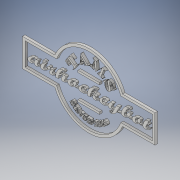
# Autodesk Inventor part: Emblem_script
Saved by Autodesk Inventor 2019.3 (Build 233278000, 278)
## iProperties
Created: 2020-09-20
Part Number: Emblem_script
Material: Generisch
Document SubType Name: Modeling
Designer: Nicolas Frick
Density: 1 g/cm^3
Appearance: Vorgabe
Author: Nicolas Frick
Autodesk Inventor part; units mm, degrees
(part 1 of 2)
ref_plane "YZ Plane" through (0, 0, 0) normal (1, 0, 0) x (0, 1, 0)
ref_plane "XZ Plane" through (0, 0, 0) normal (0, 1, 0) x (-1, 0, 0)
sketch "Skizze1" plane through (0, 0, 0) normal (0, 0, 1) x (1, 0, 0)
  line L0 (-50, 9) -> (-50, -9) construction
  line L1 (50, 9) -> (50, -9) construction
  line L2 (-50, -9) -> (-50, 9)
  line L3 (-50, 9) -> (-25.1982, 9)
  line L4 (25.1982, 9) -> (50, 9)
  line L5 (50, -9) -> (25.1982, -9)
  line L6 (-25.1982, -9) -> (-50, -9)
  line L7 (50, 9) -> (29.5255, 5.3146) construction
  arc A0 (25.1982, 9) -> (-25.1982, 9) centre (0, 0) ccw
  arc A1 (-25.1982, -9) -> (25.1982, -9) centre (0, 0) ccw
  line L8 (50, -12.5) -> (50, -9) construction
  line L9 (50, 9) -> (50, 12.5) construction
  line L10 (50, 9) -> (50, -9)
  point P0 (0, 0)
  dimension "d13" = 100
  dimension "d14" = 18
  constraints: 22 end point, 7 parallel, 4 point on circle, 2 centre point, 2 horizontal, 2 perpendicular, 1 coincident, 1 collinear
  measures "d13" distance of L0.end L1.end
  measures "d14" distance of L1.start L1.end
ref_plane "Arbeitsebene3" through (0, 0, 0) normal (0, 0, -1) x (-1, 0, 0)
sketch "Skizze3" plane through (0, 0, 0) normal (0, 0, -1) x (-1, 0, 0)
  line L0 (50, -12.5) -> (50, 12.5) construction
  line L1 (50, 12.5) -> (27.2718, 12.5) construction
  arc A0 (27.2718, 12.5) -> (-27.2718, 12.5) centre (0, 0) ccw construction
  line L2 (-27.2718, 12.5) -> (-50, 12.5) construction
  line L3 (-50, 12.5) -> (-50, -12.5) construction
  line L4 (-50, -12.5) -> (-27.2718, -12.5) construction
  arc A1 (-27.2718, -12.5) -> (27.2718, -12.5) centre (0, 0) ccw construction
  line L5 (27.2718, -12.5) -> (50, -12.5) construction
  line L6 (50, 9) -> (50, -9) projected
  line L7 (50, -9) -> (25.1982, -9) projected
  arc A2 (-25.1982, -9) -> (25.1982, -9) centre (0, 0) ccw projected
  line L8 (-25.1982, -9) -> (-50, -9) projected
  line L9 (-50, -9) -> (-50, 9) projected
  line L10 (-50, 9) -> (-25.1982, 9) projected
  arc A3 (25.1982, 9) -> (-25.1982, 9) centre (0, 0) ccw projected
  line L11 (25.1982, 9) -> (50, 9) projected
  line L12 (-26.5702, 11) -> (-52, 11)
  line L13 (-52, 11) -> (-52, -11)
  line L14 (-52, -11) -> (-26.5702, -11)
  arc A4 (-26.5702, -11) -> (26.5702, -11) centre (0, 0) ccw
  line L15 (26.5702, -11) -> (52, -11)
  line L16 (52, -11) -> (52, 11)
  line L17 (52, 11) -> (26.5702, 11)
  arc A5 (26.5702, 11) -> (-26.5702, 11) centre (0, 0) ccw
  dimension "d15" = 2
  constraints: 12 end point, 4 point on circle, 2 centre point, 7 other
  measures "d15" radial gap between concentric circles of A3 A5
ref_plane "Arbeitsebene2" through (0, 0, 3) normal (0, 0, 1) x (1, 0, 0)
sketch "Skizze4" plane through (0, 0, 3) normal (0, 0, 1) x (1, 0, 0)
  arc A0 (27.2718, 12.5) -> (-27.2718, 12.5) centre (0, 0) ccw construction
  arc A1 (14.0689, 14.5714) -> (-13.3793, 13.406) centre (0.8375, 2.3845) ccw construction
  line L0 (-50, 9) -> (-50, -9) projected
  line L1 (-48.0831, -3.7083) -> (51.9405, -3.7083) construction
  line L2 (-0.0067, -3.7083) -> (-47.5067, -3.7083) construction
  line L3 (-47.5067, -3.7083) -> (47.4933, -3.7083) construction
  arc A2 (-13.3793, -16.6178) -> (14.0689, -16.6178) centre (0.3448, -2.5459) ccw construction
  spline S0 degree 2 poles (-37.8675, -2.4944) (-39.3666, -3.3302) (-40.6602, -3.8343) (-41.2506, -3.8343) knots 0 0 0 1 2 2 2
  spline S1 degree 2 poles (-41.2506, -3.8343) (-42.7365, -3.8343) (-42.6502, -2.2953) knots 0 0 0 1 1 1
  spline S2 degree 2 poles (-42.6502, -2.2953) (-43.5855, -3.0847) (-45.171, -3.8343) (-46.0134, -3.8343) knots 0 0 0 1 2 2 2
  spline S3 degree 2 poles (-46.0134, -3.8343) (-46.836, -3.8343) (-47.9902, -2.9255) (-47.9902, -2.2622) knots 0 0 0 1 2 2 2
  spline S4 degree 2 poles (-47.9902, -2.2622) (-47.9902, -1.4396) (-46.4446, 0.0595) (-44.03, 0.9882) (-43.1013, 0.9882) knots 0 0 0 1 2 3 3 3
  spline S5 degree 2 poles (-43.1013, 0.9882) (-41.9272, 0.9882) (-41.4628, 0.3514) knots 0 0 0 1 1 1
  line L4 (-41.4628, 0.3514) -> (-39.5457, 0.975)
  line L5 (-39.5457, 0.975) -> (-39.0217, 0.975)
  line L6 (-39.0217, 0.975) -> (-39.8443, -0.637)
  spline S6 degree 2 poles (-39.8443, -0.637) (-40.4877, -1.8575) (-40.4877, -2.3086) knots 0 0 0 1 1 1
  spline S7 degree 2 poles (-40.4877, -2.3086) (-40.4877, -2.7796) (-39.9106, -2.7796) knots 0 0 0 1 1 1
  spline S8 degree 2 poles (-39.9106, -2.7796) (-39.5457, -2.7796) (-38.6635, -2.3219) (-37.8675, -1.8575) knots 0 0 0 1 2 2 2
  line L7 (-37.8675, -1.8575) -> (-37.8675, -2.4944)
  spline S9 degree 2 poles (-44.7265, -2.7929) (-43.7912, -2.7929) (-42.1328, -0.9156) (-42.1328, -0.1196) knots 0 0 0 1 2 2 2
  spline S10 degree 2 poles (-42.1328, -0.1196) (-42.1328, 0.1922) (-42.6038, 0.5372) (-42.9952, 0.5372) knots 0 0 0 1 2 2 2
  spline S11 degree 2 poles (-42.9952, 0.5372) (-43.9305, 0.5372) (-45.6088, -1.3401) (-45.6088, -2.1229) knots 0 0 0 1 2 2 2
  spline S12 degree 2 poles (-45.6088, -2.1229) (-45.6088, -2.4214) (-45.1112, -2.7929) (-44.7265, -2.7929) knots 0 0 0 1 2 2 2
  spline S13 degree 2 poles (-33.1444, -2.4944) (-35.3335, -3.8476) (-36.4214, -3.8476) knots 0 0 0 1 1 1
  spline S14 degree 2 poles (-36.4214, -3.8476) (-37.025, -3.8476) (-37.8476, -3.1245) (-37.8476, -2.5806) knots 0 0 0 1 2 2 2
  spline S15 degree 2 poles (-37.8476, -2.5806) (-37.8476, -1.4065) (-36.501, 0.6698) knots 0 0 0 1 1 1
  line L8 (-36.501, 0.6698) -> (-34.1195, 0.9617)
  line L9 (-34.1195, 0.9617) -> (-34.0068, 0.9617)
  line L10 (-34.0068, 0.9617) -> (-34.9421, -0.763)
  spline S16 degree 2 poles (-34.9421, -0.763) (-35.5258, -1.831) (-35.5258, -2.2887) knots 0 0 0 1 1 1
  spline S17 degree 2 poles (-35.5258, -2.2887) (-35.5258, -2.4678) (-35.2539, -2.6934) (-35.0482, -2.6934) knots 0 0 0 1 2 2 2
  spline S18 degree 2 poles (-35.0482, -2.6934) (-34.6834, -2.6934) (-33.9404, -2.3816) (-33.1444, -1.8575) knots 0 0 0 1 2 2 2
  line L11 (-33.1444, -1.8575) -> (-33.1444, -2.4944)
  spline S19 degree 2 poles (-33.3302, 3.111) (-33.3302, 1.7909) (-34.9885, 1.7909) knots 0 0 0 1 1 1
  spline S20 degree 2 poles (-34.9885, 1.7909) (-35.7978, 1.7909) (-36.3683, 2.0761) knots 0 0 0 1 1 1
  spline S21 degree 2 poles (-36.3683, 2.0761) (-35.8244, 2.5604) (-35.5258, 3.164) knots 0 0 0 1 1 1
  spline S22 degree 2 poles (-35.5258, 3.164) (-34.7829, 2.8987) (-34.3318, 2.8987) knots 0 0 0 1 1 1
  spline S23 degree 2 poles (-34.3318, 2.8987) (-33.8277, 2.8987) (-33.3302, 3.111) knots 0 0 0 1 1 1
  spline S24 degree 2 poles (-26.0399, -2.4944) (-28.3948, -3.8476) (-29.6685, -3.8476) knots 0 0 0 1 1 1
  spline S25 degree 2 poles (-29.6685, -3.8476) (-30.2389, -3.8476) (-31.0283, -3.2771) (-31.0283, -2.8592) knots 0 0 0 1 2 2 2
  spline S26 degree 2 poles (-31.0283, -2.8592) (-31.0283, -2.0831) (-29.6154, -0.7763) knots 0 0 0 1 1 1
  spline S27 degree 2 poles (-29.6154, -0.7763) (-30.3053, -0.9885) (-31.1278, -1.0682) knots 0 0 0 1 1 1
  spline S28 degree 2 poles (-31.1278, -1.0682) (-31.7381, -1.7315) (-33.0449, -2.4944) knots 0 0 0 1 1 1
  line L12 (-33.0449, -2.4944) -> (-33.2572, -2.4944)
  line L13 (-33.2572, -2.4944) -> (-33.2572, -1.9968)
  spline S29 degree 2 poles (-33.2572, -1.9968) (-32.5275, -1.5458) (-31.9371, -1.035) knots 0 0 0 1 1 1
  spline S30 degree 2 poles (-31.9371, -1.035) (-32.7398, -0.8227) (-32.7398, -0.4114) knots 0 0 0 1 1 1
  spline S31 degree 2 poles (-32.7398, -0.4114) (-32.7398, 0.0131) (-31.758, 0.975) (-30.8957, 0.975) knots 0 0 0 1 2 2 2
  spline S32 degree 2 poles (-30.8957, 0.975) (-30.166, 0.975) (-30.166, 0.5372) knots 0 0 0 1 1 1
  spline S33 degree 2 poles (-30.166, 0.5372) (-30.166, 0.1856) (-30.5839, -0.4579) knots 0 0 0 1 1 1
  spline S34 degree 2 poles (-30.5839, -0.4579) (-29.0316, -0.3584) (-27.8708, 0.9418) knots 0 0 0 1 1 1
  line L14 (-27.8708, 0.9418) -> (-27.0151, 0.9617)
  line L15 (-27.0151, 0.9617) -> (-27.8907, -0.4512)
  spline S35 degree 2 poles (-27.8907, -0.4512) (-28.4346, -1.3401) (-28.753, -1.9836) (-28.753, -2.2356) knots 0 0 0 1 2 2 2
  spline S36 degree 2 poles (-28.753, -2.2356) (-28.753, -2.4612) (-28.3882, -2.7398) (-28.0764, -2.7398) knots 0 0 0 1 2 2 2
  spline S37 degree 2 poles (-28.0764, -2.7398) (-27.7381, -2.7398) (-27.1212, -2.4678) (-26.0399, -1.8575) knots 0 0 0 1 2 2 2
  line L16 (-26.0399, -1.8575) -> (-26.0399, -2.4944)
  spline S38 degree 2 poles (-16.6336, -2.4944) (-18.8492, -3.8476) (-20.2821, -3.8476) knots 0 0 0 1 1 1
  spline S39 degree 2 poles (-20.2821, -3.8476) (-20.9189, -3.8476) (-21.7547, -3.3368) (-21.7547, -2.9454) knots 0 0 0 1 2 2 2
  spline S40 degree 2 poles (-21.7547, -2.9454) (-21.7547, -2.2821) (-20.8923, -1.0814) knots 0 0 0 1 1 1
  spline S41 degree 2 poles (-20.8923, -1.0814) (-20.4346, -0.4313) (-20.4346, -0.2323) knots 0 0 0 1 1 1
  spline S42 degree 2 poles (-20.4346, -0.2323) (-20.4346, -0.0068) (-20.7995, -0.0068) knots 0 0 0 1 1 1
  spline S43 degree 2 poles (-20.7995, -0.0068) (-21.1776, -0.0068) (-22.6038, -0.6038) (-23.3932, -1.1212) knots 0 0 0 1 2 2 2
  spline S44 degree 2 poles (-23.3932, -1.1212) (-23.7182, -2.1361) (-23.7182, -3.5623) knots 0 0 0 1 1 1
  line L17 (-23.7182, -3.5623) -> (-25.8078, -3.8476)
  spline S45 degree 2 poles (-25.8078, -3.8476) (-25.9272, -3.2705) (-25.9272, -2.5939) knots 0 0 0 1 1 1
  spline S46 degree 2 poles (-25.9272, -2.5939) (-25.9272, -0.9487) (-24.3882, 1.8838) (-22.7431, 3.4692) knots 0 0 0 1 2 2 2
  spline S47 degree 2 poles (-22.7431, 3.4692) (-21.5159, 3.761) (-19.685, 4.1325) (-19.559, 4.1325) knots 0 0 0 1 2 2 2
  spline S48 degree 2 poles (-19.559, 4.1325) (-19.3136, 4.1325) (-18.9753, 3.6682) (-18.9753, 3.3232) knots 0 0 0 1 2 2 2
  spline S49 degree 2 poles (-18.9753, 3.3232) (-18.9753, 2.7395) (-20.1958, 1.3199) (-21.496, 0.3183) knots 0 0 0 1 2 2 2
  spline S50 degree 2 poles (-21.496, 0.3183) (-20.2489, 0.7428) (-19.4197, 0.9617) (-18.9885, 0.9617) knots 0 0 0 1 2 2 2
  spline S51 degree 2 poles (-18.9885, 0.9617) (-18.5109, 0.9617) (-17.9139, 0.5571) (-17.9139, 0.2254) knots 0 0 0 1 2 2 2
  spline S52 degree 2 poles (-17.9139, 0.2254) (-17.9139, -0.2721) (-19.2605, -2.3484) (-19.2605, -2.6138) knots 0 0 0 1 2 2 2
  spline S53 degree 2 poles (-19.2605, -2.6138) (-19.2605, -2.7332) (-19.0084, -2.9189) (-18.8426, -2.9189) knots 0 0 0 1 2 2 2
  spline S54 degree 2 poles (-18.8426, -2.9189) (-18.2456, -2.9189) (-16.6336, -1.8575) knots 0 0 0 1 1 1
  line L18 (-16.6336, -1.8575) -> (-16.6336, -2.4944)
  spline S55 degree 2 poles (-23.1278, -0.2323) (-19.7779, 2.0562) (-19.7779, 3.1375) knots 0 0 0 1 1 1
  spline S56 degree 2 poles (-19.7779, 3.1375) (-19.7779, 3.4692) (-20.0897, 3.4692) knots 0 0 0 1 1 1
  spline S57 degree 2 poles (-20.0897, 3.4692) (-20.6005, 3.4692) (-22.5176, 1.3) (-23.1278, -0.2323) knots 0 0 0 1 2 2 2
  spline S58 degree 2 poles (-8.1229, -2.4944) (-8.6005, -2.7398) (-9.5026, -2.9388) (-9.7613, -2.9388) knots 0 0 0 1 2 2 2
  spline S59 degree 2 poles (-9.7613, -2.9388) (-10.4379, -2.9388) (-11.1013, -2.6337) knots 0 0 0 1 1 1
  spline S60 degree 2 poles (-11.1013, -2.6337) (-12.4545, -3.8343) (-14.1991, -3.8343) knots 0 0 0 1 1 1
  spline S61 degree 2 poles (-14.1991, -3.8343) (-15.2804, -3.8343) (-16.6336, -2.8725) (-16.6336, -2.0831) knots 0 0 0 1 2 2 2
  spline S62 degree 2 poles (-16.6336, -2.0831) (-16.6336, -0.8293) (-13.5955, 0.975) (-11.486, 0.975) knots 0 0 0 1 2 2 2
  spline S63 degree 2 poles (-11.486, 0.975) (-10.69, 0.975) (-9.9471, 0.7693) (-9.7812, 0.4974) (-9.7812, 0.2851) knots 0 0 0 1 2 3 3 3
  spline S64 degree 2 poles (-9.7812, 0.2851) (-9.7812, -0.7431) (-10.7365, -2.2423) knots 0 0 0 1 1 1
  spline S65 degree 2 poles (-10.7365, -2.2423) (-10.2588, -2.501) (-9.7348, -2.501) knots 0 0 0 1 1 1
  spline S66 degree 2 poles (-9.7348, -2.501) (-9.1046, -2.501) (-8.1229, -1.8575) knots 0 0 0 1 1 1
  line L19 (-8.1229, -1.8575) -> (-8.1229, -2.4944)
  spline S67 degree 2 poles (-11.2141, 0.5902) (-11.3534, 0.6234) (-11.6187, 0.6234) knots 0 0 0 1 1 1
  spline S68 degree 2 poles (-11.6187, 0.6234) (-12.8393, 0.6234) (-14.219, -0.8758) (-14.219, -1.8774) knots 0 0 0 1 2 2 2
  spline S69 degree 2 poles (-14.219, -1.8774) (-14.219, -2.4347) (-13.6154, -3.0516) (-13.0847, -3.0516) knots 0 0 0 1 2 2 2
  spline S70 degree 2 poles (-13.0847, -3.0516) (-12.4147, -3.0516) (-11.6386, -2.3285) knots 0 0 0 1 1 1
  spline S71 degree 2 poles (-11.6386, -2.3285) (-12.5142, -1.6784) (-12.5142, -0.9288) knots 0 0 0 1 1 1
  spline S72 degree 2 poles (-12.5142, -0.9288) (-12.5142, -0.0466) (-11.2141, 0.5902) knots 0 0 0 1 1 1
  spline S73 degree 2 poles (-1.0184, -2.4944) (-2.219, -3.1842) (-4.2157, -3.8343) (-5.3036, -3.8343) knots 0 0 0 1 2 2 2
  spline S74 degree 2 poles (-5.3036, -3.8343) (-6.5176, -3.8343) (-8.103, -2.9056) (-8.103, -2.1892) knots 0 0 0 1 2 2 2
  spline S75 degree 2 poles (-8.103, -2.1892) (-8.103, -1.0151) (-5.1909, 0.975) (-3.4927, 0.975) knots 0 0 0 1 2 2 2
  spline S76 degree 2 poles (-3.4927, 0.975) (-2.6569, 0.975) (-1.6088, 0.431) (-1.6088, -0.0068) knots 0 0 0 1 2 2 2
  spline S77 degree 2 poles (-1.6088, -0.0068) (-1.6088, -0.1594) (-1.8078, -0.3119) (-2.0797, -0.3915) knots 0 0 0 1 2 2 2
  line L20 (-2.0797, -0.3915) -> (-3.161, -0.6967)
  spline S78 degree 2 poles (-3.161, -0.6967) (-3.36, -0.7497) (-3.4529, -0.7497) knots 0 0 0 1 1 1
  spline S79 degree 2 poles (-3.4529, -0.7497) (-3.5855, -0.7497) (-3.5855, -0.637) knots 0 0 0 1 1 1
  spline S80 degree 2 poles (-3.5855, -0.637) (-3.5855, -0.5972) (-3.4728, -0.1063) (-3.4728, -0.0466) knots 0 0 0 1 2 2 2
  spline S81 degree 2 poles (-3.4728, -0.0466) (-3.4728, 0.1922) (-3.8177, 0.4907) (-4.1096, 0.4907) knots 0 0 0 1 2 2 2
  spline S82 degree 2 poles (-4.1096, 0.4907) (-4.7928, 0.4907) (-5.9272, -0.6967) (-5.9272, -1.4595) knots 0 0 0 1 2 2 2
  spline S83 degree 2 poles (-5.9272, -1.4595) (-5.9272, -2.1162) (-4.8592, -2.899) (-3.9703, -2.899) knots 0 0 0 1 2 2 2
  spline S84 degree 2 poles (-3.9703, -2.899) (-3.2074, -2.899) (-1.8741, -2.3882) (-1.0184, -1.8575) knots 0 0 0 1 2 2 2
  line L21 (-1.0184, -1.8575) -> (-1.0184, -2.4944)
  spline S85 degree 2 poles (8.2553, -2.4811) (6.1325, -3.8476) (4.7262, -3.8476) knots 0 0 0 1 1 1
  spline S86 degree 2 poles (4.7262, -3.8476) (4.0496, -3.8476) (3.1342, -3.2904) (3.1342, -2.8857) knots 0 0 0 1 2 2 2
  spline S87 degree 2 poles (3.1342, -2.8857) (3.1342, -2.6934) (3.3597, -1.9172) (3.3597, -1.8708) knots 0 0 0 1 2 2 2
  spline S88 degree 2 poles (3.3597, -1.8708) (3.3597, -1.6121) (2.3846, -1.5988) (2.3846, -1.3866) knots 0 0 0 1 2 2 2
  spline S89 degree 2 poles (2.3846, -1.3866) (2.3846, -1.1942) (2.6566, -1.0483) (3.0281, -1.0483) knots 0 0 0 1 2 2 2
  spline S90 degree 2 poles (3.0281, -1.0483) (4.0629, -1.0284) (5.0712, -0.564) (5.0712, -0.239) knots 0 0 0 1 2 2 2
  spline S91 degree 2 poles (5.0712, -0.239) (5.0712, -0.0134) (4.5206, 0.2784) (4.0894, 0.2784) knots 0 0 0 1 2 2 2
  spline S92 degree 2 poles (4.0894, 0.2784) (3.8506, 0.2784) (3.6383, 0.2453) knots 0 0 0 1 1 1
  spline S93 degree 2 poles (3.6383, 0.2453) (3.4128, 0.2121) (3.2072, 0.1458) knots 0 0 0 1 1 1
  spline S94 degree 2 poles (3.2072, 0.1458) (2.9883, 0.0728) (2.7561, -0.0333) knots 0 0 0 1 1 1
  spline S95 degree 2 poles (2.7561, -0.0333) (2.5305, -0.1527) (2.2785, -0.3186) knots 0 0 0 1 1 1
  spline S96 degree 2 poles (2.2785, -0.3186) (2.033, -0.4778) (1.7478, -0.6967) knots 0 0 0 1 1 1
  spline S97 degree 2 poles (1.7478, -0.6967) (1.5952, -0.8161) (1.3697, -1.7846) knots 0 0 0 1 1 1
  spline S98 degree 2 poles (1.3697, -1.7846) (1.2569, -2.2887) (1.2171, -2.7133) knots 0 0 0 1 1 1
  spline S99 degree 2 poles (1.2171, -2.7133) (1.1839, -3.1113) (1.2105, -3.6088) knots 0 0 0 1 1 1
  line L22 (1.2105, -3.6088) -> (-0.9189, -3.8211)
  spline S100 degree 2 poles (-0.9189, -3.8211) (-1.0383, -3.4031) (-1.0383, -2.7929) knots 0 0 0 1 1 1
  spline S101 degree 2 poles (-1.0383, -2.7929) (-1.0383, -1.1411) (0.4808, 1.8705) (2.2055, 3.4559) knots 0 0 0 1 2 2 2
  spline S102 degree 2 poles (2.2055, 3.4559) (3.5455, 3.7743) (5.4891, 4.1325) (5.6019, 4.1325) knots 0 0 0 1 2 2 2
  spline S103 degree 2 poles (5.6019, 4.1325) (5.8274, 4.1325) (6.2586, 3.6018) (6.2586, 3.31) knots 0 0 0 1 2 2 2
  spline S104 degree 2 poles (6.2586, 3.31) (6.2586, 2.8191) (5.1508, 1.6582) (3.9899, 0.8357) knots 0 0 0 1 2 2 2
  spline S105 degree 2 poles (3.9899, 0.8357) (4.7859, 0.975) (5.3166, 0.975) knots 0 0 0 1 1 1
  spline S106 degree 2 poles (5.3166, 0.975) (6.1856, 0.975) (7.2934, 0.4509) (7.2934, 0.0463) knots 0 0 0 1 2 2 2
  spline S107 degree 2 poles (7.2934, 0.0463) (7.2934, -0.8691) (4.4941, -1.2937) knots 0 0 0 1 1 1
  spline S108 degree 2 poles (4.4941, -1.2937) (5.5886, -1.4463) (5.5886, -2.0499) knots 0 0 0 1 1 1
  line L23 (5.5886, -2.0499) -> (5.5355, -2.5474)
  spline S109 degree 2 poles (5.5355, -2.5474) (5.5355, -2.8857) (6.0662, -2.8857) knots 0 0 0 1 1 1
  spline S110 degree 2 poles (6.0662, -2.8857) (6.4443, -2.8857) (7.3929, -2.4546) (8.2553, -1.8443) knots 0 0 0 1 2 2 2
  line L24 (8.2553, -1.8443) -> (8.2553, -2.4811)
  line L25 (2.1126, 0.1789) -> (2.7295, 0.577)
  spline S111 degree 2 poles (2.7295, 0.577) (5.4692, 2.3945) (5.4692, 3.1441) knots 0 0 0 1 1 1
  spline S112 degree 2 poles (5.4692, 3.1441) (5.4692, 3.4824) (4.965, 3.4824) knots 0 0 0 1 1 1
  spline S113 degree 2 poles (4.965, 3.4824) (4.3813, 3.4824) (2.8755, 1.8705) (2.1126, 0.1789) knots 0 0 0 1 2 2 2
  spline S114 degree 2 poles (15.3597, -2.4944) (14.1723, -3.1776) (12.2752, -3.8343) (11.1342, -3.8343) knots 0 0 0 1 2 2 2
  spline S115 degree 2 poles (11.1342, -3.8343) (9.8606, -3.8343) (8.2951, -2.8791) (8.2951, -2.0963) knots 0 0 0 1 2 2 2
  spline S116 degree 2 poles (8.2951, -2.0963) (8.2951, -0.9288) (11.048, 0.9617) (12.7262, 0.9617) knots 0 0 0 1 2 2 2
  spline S117 degree 2 poles (12.7262, 0.9617) (13.6019, 0.9617) (14.6499, 0.431) (14.6499, 0.0065) knots 0 0 0 1 2 2 2
  spline S118 degree 2 poles (14.6499, 0.0065) (14.6499, -1.1345) (10.5239, -1.8443) knots 0 0 0 1 1 1
  spline S119 degree 2 poles (10.5239, -1.8443) (10.902, -2.9189) (12.4808, -2.9189) knots 0 0 0 1 1 1
  spline S120 degree 2 poles (12.4808, -2.9189) (13.1043, -2.9189) (14.2254, -2.5275) (15.3597, -1.8575) knots 0 0 0 1 2 2 2
  line L26 (15.3597, -1.8575) -> (15.3597, -2.4944)
  spline S121 degree 2 poles (10.4509, -1.4728) (12.8523, -1.0748) (12.8523, -0.0068) knots 0 0 0 1 1 1
  spline S122 degree 2 poles (12.8523, -0.0068) (12.8523, 0.5239) (12.1956, 0.5239) knots 0 0 0 1 1 1
  spline S123 degree 2 poles (12.1956, 0.5239) (11.5786, 0.5239) (10.4509, -0.5839) (10.4509, -1.4728) knots 0 0 0 1 2 2 2
  spline S124 degree 2 poles (25.4227, -2.4944) (24.2354, -3.171) (21.6151, -3.8741) knots 0 0 0 1 1 1
  spline S125 degree 2 poles (21.6151, -3.8741) (20.7461, -5.3335) (18.5703, -6.5408) (17.3896, -6.5408) knots 0 0 0 1 2 2 2
  spline S126 degree 2 poles (17.3896, -6.5408) (16.7926, -6.5408) (16.0695, -6.1096) (16.0695, -5.7514) knots 0 0 0 1 2 2 2
  spline S127 degree 2 poles (16.0695, -5.7514) (16.0695, -4.6635) (19.4526, -3.7813) knots 0 0 0 1 1 1
  line L27 (19.4526, -3.7813) -> (20.0231, -2.6005)
  spline S128 degree 2 poles (20.0231, -2.6005) (18.2519, -3.7614) (16.912, -3.7614) knots 0 0 0 1 1 1
  spline S129 degree 2 poles (16.912, -3.7614) (16.1889, -3.7614) (15.3, -3.0648) (15.3, -2.4877) knots 0 0 0 1 2 2 2
  spline S130 degree 2 poles (15.3, -2.4877) (15.3, -1.6585) (15.9169, -0.7033) knots 0 0 0 1 1 1
  line L28 (15.9169, -0.7033) -> (16.8191, 0.6964)
  line L29 (16.8191, 0.6964) -> (19.5388, 0.975)
  line L30 (19.5388, 0.975) -> (18.3713, -0.6635)
  spline S131 degree 2 poles (18.3713, -0.6635) (17.5687, -1.8443) (17.5687, -2.4413) knots 0 0 0 1 1 1
  spline S132 degree 2 poles (17.5687, -2.4413) (17.5687, -2.9388) (18.1392, -2.9388) knots 0 0 0 1 1 1
  spline S133 degree 2 poles (18.1392, -2.9388) (18.7229, -2.9388) (20.2088, -1.8376) (20.7196, -1.035) knots 0 0 0 1 2 2 2
  line L31 (20.7196, -1.035) -> (21.7876, 0.6964)
  line L32 (21.7876, 0.6964) -> (24.3415, 0.975)
  line L33 (24.3415, 0.975) -> (21.907, -3.3302)
  spline S134 degree 2 poles (21.907, -3.3302) (24.0496, -2.7531) (25.4227, -1.8575) knots 0 0 0 1 1 1
  line L34 (25.4227, -1.8575) -> (25.4227, -2.4944)
  spline S135 degree 2 poles (19.1806, -4.3318) (18.0264, -4.6303) (16.7793, -5.3866) (16.7793, -5.7514) knots 0 0 0 1 2 2 2
  spline S136 degree 2 poles (16.7793, -5.7514) (16.7793, -6.1229) (17.3166, -6.1229) knots 0 0 0 1 1 1
  spline S137 degree 2 poles (17.3166, -6.1229) (18.3581, -6.1229) (19.1806, -4.3318) knots 0 0 0 1 1 1
  spline S138 degree 2 poles (33.9534, -2.4944) (33.3033, -2.899) (32.3747, -2.899) knots 0 0 0 1 1 1
  spline S139 degree 2 poles (32.3747, -2.899) (31.645, -2.899) (30.8224, -2.4944) knots 0 0 0 1 1 1
  spline S140 degree 2 poles (30.8224, -2.4944) (29.8208, -3.171) (28.2752, -3.8211) (27.3664, -3.8211) knots 0 0 0 1 2 2 2
  spline S141 degree 2 poles (27.3664, -3.8211) (26.5504, -3.8211) (25.4426, -3.025) (25.4426, -2.4347) knots 0 0 0 1 2 2 2
  spline S142 degree 2 poles (25.4426, -2.4347) (25.4426, -1.2871) (27.7312, 2.6267) (28.8257, 3.6284) knots 0 0 0 1 2 2 2
  spline S143 degree 2 poles (28.8257, 3.6284) (30.0596, 3.8605) (31.9435, 4.1458) (32.0828, 4.1458) knots 0 0 0 1 2 2 2
  spline S144 degree 2 poles (32.0828, 4.1458) (32.3548, 4.1458) (32.7594, 3.7212) (32.7594, 3.4227) knots 0 0 0 1 2 2 2
  spline S145 degree 2 poles (32.7594, 3.4227) (32.7594, 2.8058) (31.0214, 1.1474) (29.635, 0.3249) knots 0 0 0 1 2 2 2
  line L35 (29.635, 0.3249) -> (28.4078, -0.3982)
  spline S146 degree 2 poles (28.4078, -0.3982) (27.8241, -1.5922) (27.8241, -2.1627) knots 0 0 0 1 1 1
  spline S147 degree 2 poles (27.8241, -2.1627) (27.8241, -2.4745) (28.3083, -2.8526) (28.7063, -2.8526) knots 0 0 0 1 2 2 2
  spline S148 degree 2 poles (28.7063, -2.8526) (29.164, -2.8526) (29.9004, -2.5076) (30.3647, -2.156) knots 0 0 0 1 2 2 2
  spline S149 degree 2 poles (30.3647, -2.156) (29.8937, -1.6784) (29.8937, -1.1809) knots 0 0 0 1 1 1
  spline S150 degree 2 poles (29.8937, -1.1809) (29.8937, -0.3849) (31.3664, 0.975) (32.1956, 0.975) knots 0 0 0 1 2 2 2
  spline S151 degree 2 poles (32.1956, 0.975) (32.5272, 0.975) (32.9451, 0.63) (32.9451, 0.3514) knots 0 0 0 1 2 2 2
  spline S152 degree 2 poles (32.9451, 0.3514) (32.9451, -0.5507) (31.2204, -2.1229) knots 0 0 0 1 1 1
  spline S153 degree 2 poles (31.2204, -2.1229) (31.7378, -2.4944) (32.3946, -2.4944) knots 0 0 0 1 1 1
  spline S154 degree 2 poles (32.3946, -2.4944) (32.8058, -2.4944) (33.4095, -2.2688) (33.9534, -1.8575) knots 0 0 0 1 2 2 2
  line L36 (33.9534, -1.8575) -> (33.9534, -2.4944)
  spline S155 degree 2 poles (28.8788, 0.4642) (30.3912, 1.3398) (31.9567, 2.8191) (31.9567, 3.1972) knots 0 0 0 1 2 2 2
  spline S156 degree 2 poles (31.9567, 3.1972) (31.9567, 3.3498) (31.7246, 3.5488) (31.5521, 3.5488) knots 0 0 0 1 2 2 2
  spline S157 degree 2 poles (31.5521, 3.5488) (30.4576, 3.5488) (28.8788, 0.4642) knots 0 0 0 1 1 1
  spline S158 degree 2 poles (42.4642, -2.4944) (41.9866, -2.7398) (41.0844, -2.9388) (40.8257, -2.9388) knots 0 0 0 1 2 2 2
  spline S159 degree 2 poles (40.8257, -2.9388) (40.1491, -2.9388) (39.4858, -2.6337) knots 0 0 0 1 1 1
  spline S160 degree 2 poles (39.4858, -2.6337) (38.1325, -3.8343) (36.3879, -3.8343) knots 0 0 0 1 1 1
  spline S161 degree 2 poles (36.3879, -3.8343) (35.3067, -3.8343) (33.9534, -2.8725) (33.9534, -2.0831) knots 0 0 0 1 2 2 2
  spline S162 degree 2 poles (33.9534, -2.0831) (33.9534, -0.8293) (36.9916, 0.975) (39.101, 0.975) knots 0 0 0 1 2 2 2
  spline S163 degree 2 poles (39.101, 0.975) (39.897, 0.975) (40.64, 0.7693) (40.8058, 0.4974) (40.8058, 0.2851) knots 0 0 0 1 2 3 3 3
  spline S164 degree 2 poles (40.8058, 0.2851) (40.8058, -0.7431) (39.8506, -2.2423) knots 0 0 0 1 1 1
  spline S165 degree 2 poles (39.8506, -2.2423) (40.3282, -2.501) (40.8523, -2.501) knots 0 0 0 1 1 1
  spline S166 degree 2 poles (40.8523, -2.501) (41.4825, -2.501) (42.4642, -1.8575) knots 0 0 0 1 1 1
  line L37 (42.4642, -1.8575) -> (42.4642, -2.4944)
  spline S167 degree 2 poles (39.373, 0.5902) (39.2337, 0.6234) (38.9684, 0.6234) knots 0 0 0 1 1 1
  spline S168 degree 2 poles (38.9684, 0.6234) (37.7478, 0.6234) (36.368, -0.8758) (36.368, -1.8774) knots 0 0 0 1 2 2 2
  spline S169 degree 2 poles (36.368, -1.8774) (36.368, -2.4347) (36.9717, -3.0516) (37.5024, -3.0516) knots 0 0 0 1 2 2 2
  spline S170 degree 2 poles (37.5024, -3.0516) (38.1723, -3.0516) (38.9485, -2.3285) knots 0 0 0 1 1 1
  spline S171 degree 2 poles (38.9485, -2.3285) (38.0728, -1.6784) (38.0728, -0.9288) knots 0 0 0 1 1 1
  spline S172 degree 2 poles (38.0728, -0.9288) (38.0728, -0.0466) (39.373, 0.5902) knots 0 0 0 1 1 1
  spline S173 degree 2 poles (47.9501, -2.4944) (46.7693, -3.1776) (45.0513, -3.8343) (44.2685, -3.8343) knots 0 0 0 1 2 2 2
  spline S174 degree 2 poles (44.2685, -3.8343) (43.4659, -3.8343) (42.4642, -3.0383) (42.4642, -2.3882) knots 0 0 0 1 2 2 2
  spline S175 degree 2 poles (42.4642, -2.3882) (42.4642, -1.8111) (42.9418, -0.8758) knots 0 0 0 1 1 1
  line L38 (42.9418, -0.8758) -> (43.3531, -0.04)
  line L39 (43.3531, -0.04) -> (42.6234, -0.0599)
  line L40 (42.6234, -0.0599) -> (42.9219, 0.8025)
  line L41 (42.9219, 0.8025) -> (43.8174, 0.8224)
  line L42 (43.8174, 0.8224) -> (44.6931, 2.5405)
  line L43 (44.6931, 2.5405) -> (47.2138, 2.8456)
  line L44 (47.2138, 2.8456) -> (46.2387, 0.9285)
  line L45 (46.2387, 0.9285) -> (47.5455, 0.975)
  line L46 (47.5455, 0.975) -> (47.2403, 0.1259)
  line L47 (47.2403, 0.1259) -> (45.8009, 0.0595)
  line L48 (45.8009, 0.0595) -> (45.1707, -1.1743)
  spline S176 degree 2 poles (45.1707, -1.1743) (44.8456, -1.8177) (44.8456, -2.1958) knots 0 0 0 1 1 1
  spline S177 degree 2 poles (44.8456, -2.1958) (44.8456, -2.4546) (45.2834, -2.7796) (45.6284, -2.7796) knots 0 0 0 1 2 2 2
  spline S178 degree 2 poles (45.6284, -2.7796) (46.106, -2.7796) (47.0413, -2.4214) (47.9501, -1.8575) knots 0 0 0 1 2 2 2
  line L49 (47.9501, -1.8575) -> (47.9501, -2.4944)
  line L50 (-18.6778, 11.1239) -> (-13.9569, 17.8307)
  line L51 (-13.9569, 17.8307) -> (-11.0519, 15.7859)
  line L52 (-11.0519, 15.7859) -> (-11.133, 15.6504)
  spline S179 degree 2 poles (-11.133, 15.6504) (-12.2993, 16.3144) (-13.4711, 16.3117) knots 0 0 0 1 1 1
  spline S180 degree 2 poles (-13.4711, 16.3117) (-14.8183, 16.2827) (-15.5268, 15.2762) knots 0 0 0 1 1 1
  line L53 (-15.5268, 15.2762) -> (-15.7383, 14.9757)
  line L54 (-15.7383, 14.9757) -> (-11.3688, 11.9001)
  spline S181 degree 2 poles (-11.3688, 11.9001) (-10.329, 11.1682) (-9.6004, 12.2033) knots 0 0 0 1 1 1
  line L55 (-9.6004, 12.2033) -> (-8.9893, 13.0714)
  line L56 (-8.9893, 13.0714) -> (-8.8271, 12.9573)
  line L57 (-8.8271, 12.9573) -> (-12.3459, 7.9582)
  line L58 (-12.3459, 7.9582) -> (-12.508, 8.0723)
  line L59 (-12.508, 8.0723) -> (-11.9037, 8.931)
  spline S182 degree 2 poles (-11.9037, 8.931) (-11.1717, 9.9709) (-12.2116, 10.7028) knots 0 0 0 1 1 1
  line L60 (-12.2116, 10.7028) -> (-16.581, 13.7784)
  line L61 (-16.581, 13.7784) -> (-16.8396, 13.4111)
  spline S183 degree 2 poles (-16.8396, 13.4111) (-17.5615, 12.3855) (-17.0526, 11.0714) knots 0 0 0 1 1 1
  spline S184 degree 2 poles (-17.0526, 11.0714) (-16.802, 10.4242) (-16.2674, 9.8054) knots 0 0 0 1 1 1
  spline S185 degree 2 poles (-16.2674, 9.8054) (-16.0882, 9.5937) (-15.672, 9.2222) knots 0 0 0 1 1 1
  line L62 (-15.672, 9.2222) -> (-15.7727, 9.0791)
  line L63 (-15.7727, 9.0791) -> (-18.6778, 11.1239)
  line L64 (-6.2399, 22.2929) -> (-6.0637, 22.3545)
  line L65 (-6.0637, 22.3545) -> (-1.3895, 17.5067)
  spline S186 degree 2 poles (-1.3895, 17.5067) (-1.1685, 17.2812) (-0.7259, 17.0405) (-0.2755, 17.025) (-0.0057, 17.1193) knots 0 0 0 1 2 3 3 3
  line L66 (-0.0057, 17.1193) -> (0.1705, 17.1809)
  line L67 (0.1705, 17.1809) -> (0.236, 16.9937)
  line L68 (0.236, 16.9937) -> (-3.6019, 15.6514)
  line L69 (-3.6019, 15.6514) -> (-3.6674, 15.8386)
  line L70 (-3.6674, 15.8386) -> (-3.1663, 16.0139)
  spline S187 degree 2 poles (-3.1663, 16.0139) (-2.7919, 16.1448) (-2.5162, 16.4699) (-2.5894, 16.6791) knots 0 0 0 1 2 2 2
  spline S188 degree 2 poles (-2.5894, 16.6791) (-2.6356, 16.8113) (-2.9062, 17.1431) (-3.3108, 17.5577) knots 0 0 0 1 2 2 2
  spline S189 degree 2 poles (-3.3108, 17.5577) (-3.3369, 17.5795) (-3.4382, 17.6924) (-3.4924, 17.7414) knots 0 0 0 1 2 2 2
  line L71 (-3.4924, 17.7414) -> (-3.6873, 17.9452)
  line L72 (-3.6873, 17.9452) -> (-6.4844, 16.9668)
  line L73 (-6.4844, 16.9668) -> (-6.5278, 16.4017)
  spline S190 degree 2 poles (-6.5278, 16.4017) (-6.5438, 16.1118) (-6.4552, 15.8585) knots 0 0 0 1 1 1
  spline S191 degree 2 poles (-6.4552, 15.8585) (-6.3801, 15.6438) (-5.9896, 15.3045) (-5.7583, 15.2618) knots 0 0 0 1 2 2 2
  spline S192 degree 2 poles (-5.7583, 15.2618) (-5.6047, 15.229) (-5.3837, 15.2507) (-5.1871, 15.3071) knots 0 0 0 1 2 2 2
  line L74 (-5.1871, 15.3071) -> (-5.1216, 15.1199)
  line L75 (-5.1216, 15.1199) -> (-7.8142, 14.1781)
  line L76 (-7.8142, 14.1781) -> (-7.8796, 14.3653)
  spline S193 degree 2 poles (-7.8796, 14.3653) (-7.5994, 14.5005) (-7.3025, 14.7649) (-7.1511, 15.0033) knots 0 0 0 1 2 2 2
  spline S194 degree 2 poles (-7.1511, 15.0033) (-6.7848, 15.564) (-6.6813, 16.8053) knots 0 0 0 1 1 1
  line L77 (-6.6813, 16.8053) -> (-6.2399, 22.2929)
  line L78 (-6.1998, 20.5703) -> (-6.469, 17.17)
  line L79 (-6.469, 17.17) -> (-3.8425, 18.0886)
  line L80 (-3.8425, 18.0886) -> (-6.1998, 20.5703)
  line L81 (3.1546, 23.9513) -> (5.8875, 22.9158)
  line L82 (5.8875, 22.9158) -> (6.4558, 16.974)
  line L83 (6.4558, 16.974) -> (10.8024, 21.0536)
  line L84 (10.8024, 21.0536) -> (13.3825, 20.076)
  line L85 (13.3825, 20.076) -> (13.3164, 19.9014)
  line L86 (13.3164, 19.9014) -> (13.0764, 19.9924)
  spline S195 degree 2 poles (13.0764, 19.9924) (12.4709, 20.2218) (11.6661, 19.8593) (11.4367, 19.2538) knots 0 0 0 1 2 2 2
  line L87 (11.4367, 19.2538) -> (9.994, 15.4462)
  spline S196 degree 2 poles (9.994, 15.4462) (9.7667, 14.8462) (10.1326, 14.0339) (10.7326, 13.8065) knots 0 0 0 1 2 2 2
  line L88 (10.7326, 13.8065) -> (10.9726, 13.7156)
  line L89 (10.9726, 13.7156) -> (10.9024, 13.5301)
  line L90 (10.9024, 13.5301) -> (6.6693, 15.134)
  line L91 (6.6693, 15.134) -> (6.7396, 15.3194)
  line L92 (6.7396, 15.3194) -> (7.0233, 15.212)
  spline S197 degree 2 poles (7.0233, 15.212) (7.6233, 14.9846) (8.4281, 15.3471) (8.6576, 15.9526) knots 0 0 0 1 2 2 2
  line L93 (8.6576, 15.9526) -> (10.3441, 20.4038)
  line L94 (10.3441, 20.4038) -> (10.3277, 20.41)
  line L95 (10.3277, 20.41) -> (5.3056, 15.6507)
  line L96 (5.3056, 15.6507) -> (5.1474, 15.7106)
  line L97 (5.1474, 15.7106) -> (4.4991, 22.5935)
  line L98 (4.4991, 22.5935) -> (4.4827, 22.5997)
  line L99 (4.4827, 22.5997) -> (2.885, 18.3831)
  spline S198 degree 2 poles (2.885, 18.3831) (2.7176, 17.9412) (2.8244, 17.2021) (3.3529, 16.6214) (3.8158, 16.4272) knots 0 0 0 1 2 3 3 3
  line L100 (3.8158, 16.4272) -> (3.7455, 16.2418)
  line L101 (3.7455, 16.2418) -> (0.6744, 17.4054)
  line L102 (0.6744, 17.4054) -> (0.7447, 17.5909)
  line L103 (0.7447, 17.5909) -> (0.8101, 17.5661)
  spline S199 degree 2 poles (0.8101, 17.5661) (1.4429, 17.3263) (2.444, 17.7954) (2.6838, 18.4281) knots 0 0 0 1 2 2 2
  line L104 (2.6838, 18.4281) -> (4.0562, 22.0502)
  spline S200 degree 2 poles (4.0562, 22.0502) (4.2876, 22.6611) (3.9285, 23.4584) (3.3176, 23.6899) knots 0 0 0 1 2 2 2
  line L105 (3.3176, 23.6899) -> (3.0885, 23.7767)
  line L106 (3.0885, 23.7767) -> (3.1546, 23.9513)
  line L107 (20.2209, 10.6198) -> (20.3111, 10.4698)
  line L108 (20.3111, 10.4698) -> (18.2568, 9.2337)
  line L109 (18.2568, 9.2337) -> (18.1666, 9.3837)
  spline S201 degree 2 poles (18.1666, 9.3837) (18.7439, 10.0987) (18.9593, 10.6912) knots 0 0 0 1 1 1
  spline S202 degree 2 poles (18.9593, 10.6912) (19.0988, 11.1156) (19.0845, 12.135) (18.7801, 13.218) (18.4944, 13.6929) knots 0 0 0 1 2 3 3 3
  spline S203 degree 2 poles (18.4944, 13.6929) (18.2778, 14.0527) (17.7491, 14.4903) (17.4368, 14.5679) knots 0 0 0 1 2 2 2
  spline S204 degree 2 poles (17.4368, 14.5679) (17.2157, 14.6186) (16.7765, 14.5791) (16.6166, 14.4828) knots 0 0 0 1 2 2 2
  spline S205 degree 2 poles (16.6166, 14.4828) (16.3167, 14.3024) (16.2351, 13.9401) knots 0 0 0 1 1 1
  spline S206 degree 2 poles (16.2351, 13.9401) (16.1963, 13.767) (16.237, 13.2469) (16.431, 12.5058) (16.6309, 11.8568) knots 0 0 0 1 2 3 3 3
  spline S207 degree 2 poles (16.6309, 11.8568) (16.6791, 11.6748) (16.7022, 11.6138) knots 0 0 0 1 1 1
  line L110 (16.7022, 11.6138) -> (16.7786, 11.3738)
  line L111 (16.7786, 11.3738) -> (16.8901, 10.9848)
  spline S208 degree 2 poles (16.8901, 10.9848) (17.1864, 10.0057) (17.3237, 9.0195) (17.2142, 8.5792) knots 0 0 0 1 2 2 2
  spline S209 degree 2 poles (17.2142, 8.5792) (17.1356, 8.2459) (16.7402, 7.6812) (16.4253, 7.4917) knots 0 0 0 1 2 2 2
  spline S210 degree 2 poles (16.4253, 7.4917) (16.1154, 7.3053) (15.3332, 7.2023) (14.9509, 7.3058) knots 0 0 0 1 2 2 2
  spline S211 degree 2 poles (14.9509, 7.3058) (14.4315, 7.4222) (13.5473, 8.1564) (13.1864, 8.7562) knots 0 0 0 1 2 2 2
  spline S212 degree 2 poles (13.1864, 8.7562) (12.9367, 9.1711) (12.6596, 10.0051) (12.5687, 10.6652) knots 0 0 0 1 2 2 2
  spline S213 degree 2 poles (12.5687, 10.6652) (12.5012, 11.0943) (12.3796, 11.5113) (12.2833, 11.6713) knots 0 0 0 1 2 2 2
  spline S214 degree 2 poles (12.2833, 11.6713) (12.0999, 11.9762) (11.5244, 12.2085) (11.1824, 12.0981) knots 0 0 0 1 2 2 2
  line L112 (11.1824, 12.0981) -> (11.0921, 12.248)
  line L113 (11.0921, 12.248) -> (13.8712, 13.9202)
  line L114 (13.8712, 13.9202) -> (13.9614, 13.7702)
  spline S215 degree 2 poles (13.9614, 13.7702) (13.2758, 13.2352) (12.9828, 12.3644) knots 0 0 0 1 1 1
  spline S216 degree 2 poles (12.9828, 12.3644) (12.8113, 11.846) (12.775, 10.5374) (13.0656, 9.2963) (13.3483, 8.8264) knots 0 0 0 1 2 3 3 3
  spline S217 degree 2 poles (13.3483, 8.8264) (13.598, 8.4116) (14.2879, 7.8872) (15.0123, 7.7921) (15.3222, 7.9786) knots 0 0 0 1 2 3 3 3
  spline S218 degree 2 poles (15.3222, 7.9786) (15.6471, 8.174) (15.7526, 8.5984) knots 0 0 0 1 1 1
  spline S219 degree 2 poles (15.7526, 8.5984) (15.7954, 8.7875) (15.7617, 9.2846) (15.6078, 10.0158) (15.4289, 10.6298) knots 0 0 0 1 2 3 3 3
  line L115 (15.4289, 10.6298) -> (15.2852, 11.1288)
  spline S220 degree 2 poles (15.2852, 11.1288) (14.9507, 12.2959) (14.869, 12.771) knots 0 0 0 1 1 1
  spline S221 degree 2 poles (14.869, 12.771) (14.7673, 13.302) (14.7895, 13.9894) (14.9261, 14.3167) knots 0 0 0 1 2 2 2
  spline S222 degree 2 poles (14.9261, 14.3167) (15.1066, 14.7861) (15.5215, 15.0357) knots 0 0 0 1 1 1
  spline S223 degree 2 poles (15.5215, 15.0357) (16.0163, 15.3334) (17.1689, 15.2168) (18.2543, 14.4199) (18.6423, 13.7751) knots 0 0 0 1 2 3 3 3
  spline S224 degree 2 poles (18.6423, 13.7751) (19.2318, 12.7954) (19.3215, 11.413) knots 0 0 0 1 1 1
  spline S225 degree 2 poles (19.3215, 11.413) (19.3592, 10.9318) (19.4374, 10.8019) knots 0 0 0 1 1 1
  spline S226 degree 2 poles (19.4374, 10.8019) (19.6389, 10.467) (20.2209, 10.6198) knots 0 0 0 1 1 1
  line L116 (-10.5425, -14.6538) -> (-10.422, -14.7825)
  line L117 (-10.422, -14.7825) -> (-11.3462, -15.6476)
  line L118 (-11.3462, -15.6476) -> (-11.4647, -15.521)
  spline S227 degree 2 poles (-11.4647, -15.521) (-11.2523, -15.0966) (-11.2118, -14.7973) knots 0 0 0 1 1 1
  spline S228 degree 2 poles (-11.2118, -14.7973) (-11.1888, -14.5977) (-11.2939, -14.126) (-11.5422, -13.6577) (-11.722, -13.4657) knots 0 0 0 1 2 3 3 3
  spline S229 degree 2 poles (-11.722, -13.4657) (-11.8523, -13.3264) (-12.1339, -13.1822) (-12.2788, -13.1754) knots 0 0 0 1 2 2 2
  spline S230 degree 2 poles (-12.2788, -13.1754) (-12.3809, -13.172) (-12.5628, -13.2314) (-12.6198, -13.2848) knots 0 0 0 1 2 2 2
  spline S231 degree 2 poles (-12.6198, -13.2848) (-12.7295, -13.3875) (-12.7314, -13.5674) knots 0 0 0 1 1 1
  spline S232 degree 2 poles (-12.7314, -13.5674) (-12.7333, -13.6245) (-12.6652, -13.8538) (-12.5021, -14.1802) (-12.3399, -14.4677) knots 0 0 0 1 2 3 3 3
  spline S233 degree 2 poles (-12.3399, -14.4677) (-12.2997, -14.5529) (-12.2821, -14.5759) knots 0 0 0 1 1 1
  line L119 (-12.2821, -14.5759) -> (-12.2616, -14.6359)
  line L120 (-12.2616, -14.6359) -> (-12.1277, -14.855)
  spline S234 degree 2 poles (-12.1277, -14.855) (-11.8868, -15.2985) (-11.716, -15.7642) (-11.7262, -16.0113) knots 0 0 0 1 2 2 2
  spline S235 degree 2 poles (-11.7262, -16.0113) (-11.7253, -16.1688) (-11.8669, -16.4954) (-12.002, -16.6218) knots 0 0 0 1 2 2 2
  spline S236 degree 2 poles (-12.002, -16.6218) (-12.137, -16.7482) (-12.5199, -16.8889) (-12.7404, -16.8775) knots 0 0 0 1 2 2 2
  spline S237 degree 2 poles (-12.7404, -16.8775) (-12.9917, -16.8713) (-13.5023, -16.605) (-13.7413, -16.3497) knots 0 0 0 1 2 2 2
  spline S238 degree 2 poles (-13.7413, -16.3497) (-13.9072, -16.1724) (-14.1259, -15.7992) (-14.2288, -15.5075) knots 0 0 0 1 2 2 2
  spline S239 degree 2 poles (-14.2288, -15.5075) (-14.3178, -15.294) (-14.4102, -15.1191) (-14.4675, -15.058) knots 0 0 0 1 2 2 2
  spline S240 degree 2 poles (-14.4675, -15.058) (-14.5722, -14.9461) (-14.8344, -14.8986) (-15.0012, -14.9954) knots 0 0 0 1 2 2 2
  line L121 (-15.0012, -14.9954) -> (-15.1236, -14.8645)
  line L122 (-15.1236, -14.8645) -> (-13.9041, -13.7229)
  line L123 (-13.9041, -13.7229) -> (-13.7796, -13.8558)
  spline S241 degree 2 poles (-13.7796, -13.8558) (-14.0691, -14.2021) (-14.1201, -14.6298) knots 0 0 0 1 1 1
  spline S242 degree 2 poles (-14.1201, -14.6298) (-14.1449, -14.8866) (-14.0322, -15.4976) (-13.7761, -16.0418) (-13.5983, -16.2317) knots 0 0 0 1 2 3 3 3
  spline S243 degree 2 poles (-13.5983, -16.2317) (-13.4443, -16.3963) (-13.0858, -16.5635) (-12.7639, -16.5353) (-12.6478, -16.4267) knots 0 0 0 1 2 3 3 3
  spline S244 degree 2 poles (-12.6478, -16.4267) (-12.5297, -16.316) (-12.5235, -16.1281) knots 0 0 0 1 1 1
  spline S245 degree 2 poles (-12.5235, -16.1281) (-12.5226, -16.0402) (-12.5828, -15.8195) (-12.7315, -15.4915) (-12.876, -15.2229) knots 0 0 0 1 2 3 3 3
  line L124 (-12.876, -15.2229) -> (-12.9953, -14.9982)
  spline S246 degree 2 poles (-12.9953, -14.9982) (-13.2746, -14.4757) (-13.3477, -14.275) knots 0 0 0 1 1 1
  spline S247 degree 2 poles (-13.3477, -14.275) (-13.4639, -14.0155) (-13.5261, -13.6699) (-13.4982, -13.5052) knots 0 0 0 1 2 2 2
  spline S248 degree 2 poles (-13.4982, -13.5052) (-13.4524, -13.2328) (-13.2667, -13.0589) knots 0 0 0 1 1 1
  spline S249 degree 2 poles (-13.2667, -13.0589) (-13.0494, -12.8555) (-12.4624, -12.789) (-11.8417, -13.0671) (-11.583, -13.3435) knots 0 0 0 1 2 3 3 3
  spline S250 degree 2 poles (-11.583, -13.3435) (-11.1959, -13.7571) (-11.0187, -14.3988) knots 0 0 0 1 1 1
  spline S251 degree 2 poles (-11.0187, -14.3988) (-10.9506, -14.6281) (-10.9072, -14.6745) knots 0 0 0 1 1 1
  spline S252 degree 2 poles (-10.9072, -14.6745) (-10.8045, -14.7842) (-10.5425, -14.6538) knots 0 0 0 1 1 1
  line L125 (-12.2684, -17.4028) -> (-12.151, -17.4919)
  spline S253 degree 2 poles (-12.151, -17.4919) (-11.9184, -17.6683) (-11.5337, -17.6156) (-11.352, -17.3761) knots 0 0 0 1 2 2 2
  spline S254 degree 2 poles (-11.352, -17.3761) (-11.2521, -17.2779) (-11.1189, -17.1358) (-10.9605, -16.9367) (-10.844, -16.7784) knots 0 0 0 1 2 3 3 3
  spline S255 degree 2 poles (-10.844, -16.7784) (-10.3513, -16.1147) (-10.1284, -15.7541) knots 0 0 0 1 1 1
  spline S256 degree 2 poles (-10.1284, -15.7541) (-10.0403, -15.6142) (-9.9943, -15.4387) (-10.0181, -15.3553) knots 0 0 0 1 2 2 2
  spline S257 degree 2 poles (-10.0181, -15.3553) (-10.0529, -15.1765) (-10.2693, -15.0123) knots 0 0 0 1 1 1
  line L126 (-10.2693, -15.0123) -> (-10.3867, -14.9232)
  line L127 (-10.3867, -14.9232) -> (-10.2714, -14.7712)
  line L128 (-10.2714, -14.7712) -> (-8.4825, -16.1288)
  line L129 (-8.4825, -16.1288) -> (-8.5978, -16.2807)
  line L130 (-8.5978, -16.2807) -> (-8.7152, -16.1916)
  spline S258 degree 2 poles (-8.7152, -16.1916) (-8.9478, -16.0152) (-9.3284, -16.0673) (-9.5066, -16.3022) knots 0 0 0 1 2 2 2
  line L131 (-9.5066, -16.3022) -> (-10.7017, -17.8769)
  spline S259 degree 2 poles (-10.7017, -17.8769) (-10.8799, -18.1118) (-10.8272, -18.4965) (-10.5969, -18.6712) knots 0 0 0 1 2 2 2
  line L132 (-10.5969, -18.6712) -> (-10.4795, -18.7603)
  line L133 (-10.4795, -18.7603) -> (-10.5983, -18.9169)
  line L134 (-10.5983, -18.9169) -> (-12.3872, -17.5593)
  line L135 (-12.3872, -17.5593) -> (-12.2684, -17.4028)
  line L136 (-8.802, -16.0581) -> (-7.5089, -16.6901)
  line L137 (-7.5089, -16.6901) -> (-6.5286, -19.8907)
  line L138 (-6.5286, -19.8907) -> (-5.908, -18.621)
  spline S260 degree 2 poles (-5.908, -18.621) (-5.7963, -18.3925) (-5.7833, -17.9774) (-5.8961, -17.8001) knots 0 0 0 1 2 2 2
  spline S261 degree 2 poles (-5.8961, -17.8001) (-5.938, -17.7345) (-6.0735, -17.6168) (-6.2567, -17.5112) knots 0 0 0 1 2 2 2
  line L139 (-6.2567, -17.5112) -> (-6.1742, -17.3424)
  line L140 (-6.1742, -17.3424) -> (-4.5695, -18.1267)
  line L141 (-4.5695, -18.1267) -> (-4.6533, -18.2981)
  line L142 (-4.6533, -18.2981) -> (-4.7312, -18.26)
  spline S262 degree 2 poles (-4.7312, -18.26) (-5.0376, -18.1103) (-5.5499, -18.3424) (-5.7377, -18.7267) knots 0 0 0 1 2 2 2
  line L143 (-5.7377, -18.7267) -> (-6.8279, -20.9572)
  line L144 (-6.8279, -20.9572) -> (-6.9681, -20.8887)
  line L145 (-6.9681, -20.8887) -> (-8.2125, -16.9253)
  line L146 (-8.2125, -16.9253) -> (-9.0755, -18.691)
  spline S263 degree 2 poles (-9.0755, -18.691) (-9.2024, -18.9507) (-9.2264, -19.3025) (-9.1266, -19.467) knots 0 0 0 1 2 2 2
  spline S264 degree 2 poles (-9.1266, -19.467) (-9.0624, -19.566) (-8.9103, -19.6628) knots 0 0 0 1 1 1
  spline S265 degree 2 poles (-8.9103, -19.6628) (-8.8296, -19.7215) (-8.6257, -19.8309) knots 0 0 0 1 1 1
  line L147 (-8.6257, -19.8309) -> (-8.7082, -19.9996)
  line L148 (-8.7082, -19.9996) -> (-10.3934, -19.176)
  line L149 (-10.3934, -19.176) -> (-10.3109, -19.0072)
  spline S266 degree 2 poles (-10.3109, -19.0072) (-10.0255, -19.1274) (-9.6738, -19.132) (-9.4081, -18.9306) (-9.3091, -18.728) knots 0 0 0 1 2 3 3 3
  line L150 (-9.3091, -18.728) -> (-8.4652, -17.0013)
  spline S267 degree 2 poles (-8.4652, -17.0013) (-8.3941, -16.8558) (-8.4236, -16.5937) (-8.6183, -16.3602) (-8.8001, -16.2714) knots 0 0 0 1 2 3 3 3
  line L151 (-8.8001, -16.2714) -> (-8.8858, -16.2295)
  line L152 (-8.8858, -16.2295) -> (-8.802, -16.0581)
  line L153 (-1.9582, -20.8403) -> (-1.7889, -20.8779)
  spline S268 degree 2 poles (-1.7889, -20.8779) (-1.9102, -21.1441) (-2.1151, -21.4006) (-2.2628, -21.5188) knots 0 0 0 1 2 2 2
  spline S269 degree 2 poles (-2.2628, -21.5188) (-2.9091, -22.0295) (-3.7414, -21.8447) knots 0 0 0 1 1 1
  spline S270 degree 2 poles (-3.7414, -21.8447) (-4.2634, -21.7287) (-5.0557, -21.0436) (-5.4059, -20.1013) (-5.3, -19.6244) knots 0 0 0 1 2 3 3 3
  spline S271 degree 2 poles (-5.3, -19.6244) (-5.2368, -19.3395) (-4.9011, -18.8278) (-4.3933, -18.4344) (-4.1318, -18.4036) knots 0 0 0 1 2 3 3 3
  spline S272 degree 2 poles (-4.1318, -18.4036) (-3.624, -18.1433) (-3.0964, -18.2605) knots 0 0 0 1 1 1
  spline S273 degree 2 poles (-3.0964, -18.2605) (-2.9243, -18.2987) (-2.6165, -18.4322) (-2.3622, -18.6338) (-2.2321, -18.7811) knots 0 0 0 1 2 3 3 3
  spline S274 degree 2 poles (-2.2321, -18.7811) (-2.1151, -18.9077) (-2.0531, -18.9215) knots 0 0 0 1 1 1
  spline S275 degree 2 poles (-2.0531, -18.9215) (-1.912, -18.9529) (-1.5804, -18.6594) knots 0 0 0 1 1 1
  line L154 (-1.5804, -18.6594) -> (-1.4224, -18.6945)
  line L155 (-1.4224, -18.6945) -> (-1.7278, -20.403)
  line L156 (-1.7278, -20.403) -> (-1.8971, -20.3654)
  spline S276 degree 2 poles (-1.8971, -20.3654) (-1.8981, -20.1432) (-1.9244, -19.9153) (-1.9611, -19.7739) knots 0 0 0 1 2 2 2
  spline S277 degree 2 poles (-1.9611, -19.7739) (-2.0455, -19.4206) (-2.3766, -18.8586) (-2.8306, -18.5031) (-3.0958, -18.4442) knots 0 0 0 1 2 3 3 3
  spline S278 degree 2 poles (-3.0958, -18.4442) (-3.4118, -18.374) (-3.8779, -18.6199) (-4.233, -19.2989) (-4.3602, -19.8717) knots 0 0 0 1 2 3 3 3
  spline S279 degree 2 poles (-4.3602, -19.8717) (-4.4341, -20.2046) (-4.4751, -20.7225) (-4.4093, -21.0924) (-4.3171, -21.2638) knots 0 0 0 1 2 3 3 3
  spline S280 degree 2 poles (-4.3171, -21.2638) (-4.2218, -21.3946) (-3.875, -21.6196) (-3.6437, -21.671) knots 0 0 0 1 2 2 2
  spline S281 degree 2 poles (-3.6437, -21.671) (-3.4292, -21.7186) (-3.0154, -21.695) (-2.6258, -21.5536) (-2.4531, -21.4291) knots 0 0 0 1 2 3 3 3
  spline S282 degree 2 poles (-2.4531, -21.4291) (-2.3039, -21.3172) (-2.0998, -21.0783) (-1.9582, -20.8403) knots 0 0 0 1 2 2 2
  line L157 (-1.6226, -18.6976) -> (2.097, -18.7064)
  line L158 (2.097, -18.7064) -> (2.0937, -20.1226)
  line L159 (2.0937, -20.1226) -> (1.9289, -20.1222)
  spline S283 degree 2 poles (1.9289, -20.1222) (1.82, -19.7462) (1.6676, -19.4106) (1.5841, -19.2803) knots 0 0 0 1 2 2 2
  spline S284 degree 2 poles (1.5841, -19.2803) (1.3996, -19.0891) (1.2581, -19.0194) knots 0 0 0 1 1 1
  spline S285 degree 2 poles (1.2581, -19.0194) (0.9405, -18.8944) (0.5272, -18.8934) knots 0 0 0 1 1 1
  line L160 (0.5272, -18.8934) -> (-0.0913, -18.892)
  line L161 (-0.0913, -18.892) -> (-0.0949, -20.4064)
  line L162 (-0.0949, -20.4064) -> (0.0323, -20.4067)
  spline S286 degree 2 poles (0.0323, -20.4067) (0.4051, -20.4076) (0.6284, -20.0844) knots 0 0 0 1 1 1
  spline S287 degree 2 poles (0.6284, -20.0844) (0.7445, -19.9171) (0.7999, -19.6831) knots 0 0 0 1 1 1
  spline S288 degree 2 poles (0.7999, -19.6831) (0.8291, -19.5762) (0.8586, -19.3306) knots 0 0 0 1 1 1
  line L163 (0.8586, -19.3306) -> (1.0435, -19.3311)
  line L164 (1.0435, -19.3311) -> (1.038, -21.6605)
  line L165 (1.038, -21.6605) -> (0.8559, -21.6601)
  spline S289 degree 2 poles (0.8559, -21.6601) (0.8218, -21.4404) (0.7445, -21.128) (0.6495, -20.94) (0.5718, -20.8386) knots 0 0 0 1 2 3 3 3
  spline S290 degree 2 poles (0.5718, -20.8386) (0.3729, -20.5925) (-0.0057, -20.5916) knots 0 0 0 1 1 1
  line L166 (-0.0057, -20.5916) -> (-0.0953, -20.5914)
  line L167 (-0.0953, -20.5914) -> (-0.0987, -22.0104)
  line L168 (-0.0987, -22.0104) -> (0.41, -22.0116)
  spline S291 degree 2 poles (0.41, -22.0116) (0.6528, -22.0122) (1.0402, -21.9438) (1.3411, -21.8029) (1.4744, -21.6876) knots 0 0 0 1 2 3 3 3
  spline S292 degree 2 poles (1.4744, -21.6876) (1.7032, -21.4945) (1.831, -21.2029) knots 0 0 0 1 1 1
  spline S293 degree 2 poles (1.831, -21.2029) (1.9065, -21.0354) (1.9998, -20.7062) knots 0 0 0 1 1 1
  line L169 (1.9998, -20.7062) -> (2.1819, -20.7066)
  line L170 (2.1819, -20.7066) -> (2.1783, -22.2066)
  line L171 (2.1783, -22.2066) -> (-1.6222, -22.1976)
  line L172 (-1.6222, -22.1976) -> (-1.6304, -22.0068)
  line L173 (-1.6304, -22.0068) -> (-1.4859, -22.0072)
  spline S294 degree 2 poles (-1.4859, -22.0072) (-0.9195, -22.0085) (-0.9181, -21.4334) knots 0 0 0 1 1 1
  line L174 (-0.9181, -21.4334) -> (-0.9134, -19.4565)
  spline S295 degree 2 poles (-0.9134, -19.4565) (-0.9127, -19.1617) (-1.1838, -18.8894) (-1.4786, -18.8887) knots 0 0 0 1 2 2 2
  line L175 (-1.4786, -18.8887) -> (-1.6231, -18.8883)
  line L176 (-1.6231, -18.8883) -> (-1.6226, -18.6976)
  line L177 (6.6607, -19.7285) -> (6.7941, -21.1492)
  line L178 (6.7941, -21.1492) -> (4.2209, -21.8635)
  spline S296 degree 2 poles (4.2209, -21.8635) (4.1521, -21.5616) (4.3357, -21.1747) knots 0 0 0 1 1 1
  spline S297 degree 2 poles (4.3357, -21.1747) (4.4632, -20.8994) (4.9489, -20.2936) knots 0 0 0 1 1 1
  spline S298 degree 2 poles (4.9489, -20.2936) (5.2111, -19.9629) (5.2589, -19.8867) knots 0 0 0 1 1 1
  spline S299 degree 2 poles (5.2589, -19.8867) (5.2657, -19.8788) (5.2926, -19.8353) (5.3168, -19.7926) knots 0 0 0 1 2 2 2
  spline S300 degree 2 poles (5.3168, -19.7926) (5.448, -19.5522) (5.5011, -19.1385) (5.437, -18.9074) knots 0 0 0 1 2 2 2
  spline S301 degree 2 poles (5.437, -18.9074) (5.328, -18.5147) (4.8348, -18.2077) (4.4867, -18.3043) knots 0 0 0 1 2 2 2
  spline S302 degree 2 poles (4.4867, -18.3043) (4.2166, -18.3793) (3.8265, -18.7246) (3.6731, -19.1661) (3.7342, -19.3861) knots 0 0 0 1 2 3 3 3
  spline S303 degree 2 poles (3.7342, -19.3861) (3.7921, -19.5949) (3.8562, -19.5771) knots 0 0 0 1 1 1
  spline S304 degree 2 poles (3.8562, -19.5771) (3.859, -19.5764) (3.8525, -19.5422) knots 0 0 0 1 1 1
  spline S305 degree 2 poles (3.8525, -19.5422) (3.8454, -19.4842) (3.8534, -19.4159) knots 0 0 0 1 1 1
  spline S306 degree 2 poles (3.8534, -19.4159) (3.8782, -19.2351) (4.0565, -19.0236) (4.218, -18.9788) knots 0 0 0 1 2 2 2
  spline S307 degree 2 poles (4.218, -18.9788) (4.3517, -18.9417) (4.5986, -18.9991) (4.7715, -19.1791) (4.8063, -19.3044) knots 0 0 0 1 2 3 3 3
  spline S308 degree 2 poles (4.8063, -19.3044) (4.8473, -19.452) (4.7654, -19.7297) (4.5519, -19.9329) (4.3959, -19.9762) knots 0 0 0 1 2 3 3 3
  spline S309 degree 2 poles (4.3959, -19.9762) (4.1091, -20.0559) (3.6317, -19.7624) (3.5474, -19.4589) knots 0 0 0 1 2 2 2
  spline S310 degree 2 poles (3.5474, -19.4589) (3.4972, -19.2779) (3.5398, -18.8911) (3.6651, -18.6944) knots 0 0 0 1 2 2 2
  spline S311 degree 2 poles (3.6651, -18.6944) (3.8943, -18.2558) (4.6268, -18.0525) knots 0 0 0 1 1 1
  spline S312 degree 2 poles (4.6268, -18.0525) (4.9275, -17.969) (5.4893, -17.972) (5.9433, -18.1489) (6.2525, -18.474) (6.3136, -18.694) knots 0 0 0 1 2 3 4 4 4
  spline S313 degree 2 poles (6.3136, -18.694) (6.4048, -19.0227) (6.2443, -19.3522) knots 0 0 0 1 1 1
  spline S314 degree 2 poles (6.2443, -19.3522) (6.1886, -19.4756) (6.084, -19.6066) knots 0 0 0 1 1 1
  spline S315 degree 2 poles (6.084, -19.6066) (5.9022, -19.8161) (5.5, -20.1287) knots 0 0 0 1 1 1
  spline S316 degree 2 poles (5.5, -20.1287) (4.9469, -20.5672) (4.7592, -20.8202) knots 0 0 0 1 1 1